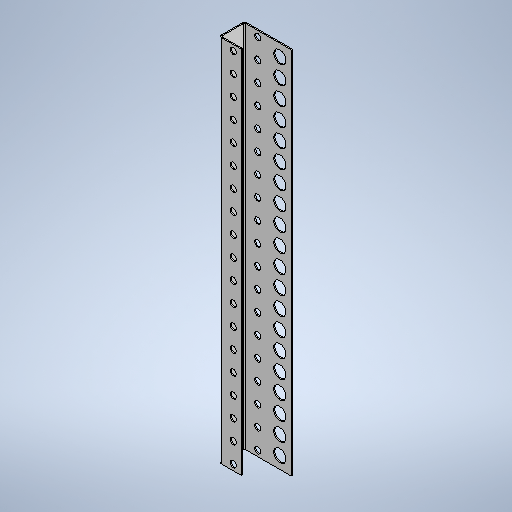
# Autodesk Inventor part: DMF 01 12 wheel pin
Saved by Autodesk Inventor 2026.2 (Build 302298010, 298A)
## iProperties
Created: 2024-04-30
Part Number: DMF 01 12 wheel pin
Material: Generic
Document SubType Name: Sheet Metal
Designer: admin
Density: 1 g/cm^3
Sheet Metal Rule: Default
Appearance: Default
Sheet Metal Width: 163,048 mm
Sheet Metal Length: 650,000 mm
Sheet Metal Area: 105981,061 mm^2
Stock Number: Барабан_Сектор_Усилителя
Flat Pattern Width: 16.3048 cm
Flat Pattern Length: 65 cm
Flat Pattern Area: 1059.81 cm^2
wheel_pin_L: 290,000 mm
wheel_pin_h: 25,000 mm
wheel_pin_Angle: 11,00 deg
Author: pokla
Autodesk Inventor part; units mm, degrees
ref_plane "YZ Plane" through (0, 0, 0) normal (1, 0, 0) x (0, 1, 0)
ref_plane "XZ Plane" through (0, 0, 0) normal (0, 1, 0) x (-1, 0, 0)
ref_plane "XY Plane" through (0, 0, 0) normal (0, 0, 1) x (1, 0, 0)
sketch "Sketch1" plane through (0, 0, 0) normal (0, 0, 1) x (1, 0, 0)
  line L0 (-42.5, 650) -> (42.5, 650)
  line L1 (42.5, 650) -> (42.5, 0)
  line L2 (42.5, 0) -> (-42.5, 0)
  line L3 (-42.5, 0) -> (-42.5, 650)
  point P0 (0, 0)
  point P1 (0, 0)
  point P2 (0, 0)
  point P3 (0, 0)
  point P4 (0, 0)
  dimension "d27" = 85
  dimension "d45" = 650
  measures "d27" distance of L1.end L2.end
  measures "d45" distance of L0.end L1.end
extrude "Plate1" add sketch "Sketch1" against normal blind 2
sketch "Sketch5" plane through (-40.5, 0, -2) normal (-1, 0, 0) x (0, -1, 0)
  line L0 (-650, 0) -> (0, 0)
  line L1 (0, 0) -> (0, 45)
  line L2 (0, 45) -> (-650, 45)
  line L3 (-650, 45) -> (-650, 0)
  constraints: 6 end point, 1 horizontal, 1 perpendicular, 1 vertical
edge flange "Flange2" height 45 angle 90 thickness 2 bend radius 2 thickness toward (-1, 0, 0) relief tear relief width 2 relief depth 1 edges at (-42.5, 325, 0) wall of the first edge with corners at (-40.5, 650, -2) (-40.5, 0, -2) (-40.5, 0, 43) (-40.5, 650, 43)
bend "Bend3"
corner "Corner2"
sketch "Sketch6" plane through (-42.5, 0, 41) normal (0, 0, 1) x (1, 0, 0)
  line L0 (0, 650) -> (0, 0)
  line L1 (0, 0) -> (40, 0)
  line L2 (40, 0) -> (40, 650)
  line L3 (40, 650) -> (0, 650)
  constraints: 6 end point, 1 horizontal, 1 perpendicular, 1 vertical
edge flange "Flange3" height 40 angle 90 thickness 2 bend radius 2 thickness toward (0, 0, 1) relief tear relief width 2 relief depth 1 edges at (-40.5, 325, 43) wall of the first edge with corners at (-42.5, 650, 41) (-42.5, 0, 41) (-2.5, 0, 41) (-2.5, 650, 41)
bend "Bend4"
corner "Corner3"
sketch "Sketch7" plane through (0, 0, 0) normal (0, 0, 1) x (1, 0, 0)
  circle A0 centre (21.5, 21.0949) radius 11
  circle A1 centre (-17.5, 10) radius 5.5
  line L0 (-38.5, 0) -> (-38.5, 650) construction
  line L1 (42.5, 650) -> (-38.5, 650) projected
  line L2 (42.5, 0) -> (42.5, 650) construction
  line L3 (-38.5, 0) -> (42.5, 0) projected
  line L4 (-38.5, 650) -> (-38.5, 0) construction
  line L5 (-2.5, 0) -> (-38.5, 0) projected
  line L6 (-2.5, 650) -> (-2.5, 0) construction
  line L7 (-38.5, 650) -> (-2.5, 650) projected
  circle A2 centre (-17.5, 45) radius 5.5
  circle A3 centre (-17.5, 80) radius 5.5
  circle A4 centre (-17.5, 115) radius 5.5
  circle A5 centre (-17.5, 150) radius 5.5
  circle A6 centre (-17.5, 185) radius 5.5
  circle A7 centre (-17.5, 220) radius 5.5
  circle A8 centre (-17.5, 255) radius 5.5
  circle A9 centre (-17.5, 290) radius 5.5
  circle A10 centre (-17.5, 325) radius 5.5
  circle A11 centre (-17.5, 360) radius 5.5
  circle A12 centre (-17.5, 395) radius 5.5
  circle A13 centre (-17.5, 430) radius 5.5
  circle A14 centre (-17.5, 465) radius 5.5
  circle A15 centre (-17.5, 500) radius 5.5
  circle A16 centre (-17.5, 535) radius 5.5
  circle A17 centre (-17.5, 570) radius 5.5
  circle A18 centre (-17.5, 605) radius 5.5
  circle A19 centre (-17.5, 640) radius 5.5
  circle A20 centre (21.5, 53.0949) radius 11
  circle A21 centre (21.5, 85.0949) radius 11
  circle A22 centre (21.5, 117.0949) radius 11
  circle A23 centre (21.5, 149.0949) radius 11
  circle A24 centre (21.5, 181.0949) radius 11
  circle A25 centre (21.5, 213.0949) radius 11
  circle A26 centre (21.5, 245.0949) radius 11
  circle A27 centre (21.5, 277.0949) radius 11
  circle A28 centre (21.5, 309.0949) radius 11
  circle A29 centre (21.5, 341.0949) radius 11
  circle A30 centre (21.5, 373.0949) radius 11
  circle A31 centre (21.5, 405.0949) radius 11
  circle A32 centre (21.5, 437.0949) radius 11
  circle A33 centre (21.5, 469.0949) radius 11
  circle A34 centre (21.5, 501.0949) radius 11
  circle A35 centre (21.5, 533.0949) radius 11
  circle A36 centre (21.5, 565.0949) radius 11
  circle A37 centre (21.5, 597.0949) radius 11
  circle A38 centre (21.5, 629.0949) radius 11
  point P0 (0, 0)
  dimension "d71" = 22
  dimension "d72" = 11
  dimension "d74" = 15
  dimension "d75" = 10
  dimension "d78" = 35
  dimension "d83" = 10
  dimension "d84" = 21
  dimension "d87" = 32
  constraints: 39 centre point, 2 vertical, 74 other
  measures "d71" diameter of A0
  measures "d72" diameter of A1
  measures "d74" distance from line of L6 A1.centre
  measures "d75" distance from line of L3 A1.centre
  measures "d78" distance of A1.centre A2.centre
  measures "d83" distance from line of A19.centre L7
  measures "d84" distance from line of L2 A0.centre
  measures "d87" distance of A0.centre A20.centre
extrude "Extrusion2" cut sketch "Sketch7" along normal through all both and the other way through all
fillet "Fillet1" radius 2 4 edges at (-2.5, 650, 42) (42.5, 650, -1) (-2.5, 0, 42) (42.5, 0, -1)
equation "\"d15\" = Thickness"
equation "\"d51\" = BendReliefWidth"
equation "\"d52\" = BendReliefDepth"
equation "\"d53\" = MinimumRemnant"
equation "\"d54\" = TransitionRadius"
equation "\"d57\" = BendRadius"
equation "\"d58\" = CornerReliefSize"
equation "\"d59\" = GapSize"
equation "\"d60\" = JacobiRadiusSize"
equation "\"d61\" = BendReliefWidth"
equation "\"d62\" = BendReliefDepth"
equation "\"d63\" = MinimumRemnant"
equation "\"d64\" = TransitionRadius"
equation "\"d67\" = BendRadius"
equation "\"d68\" = CornerReliefSize"
equation "\"d69\" = GapSize"
equation "\"d70\" = JacobiRadiusSize"
equation "\"BendRadius\" = Thickness"
equation "\"BendReliefWidth\" = Thickness"
equation "\"BendReliefDepth\" = 0.5 * Thickness"
equation "\"CornerReliefSize\" = 4 * Thickness"
equation "\"MinimumRemnant\" = 2 * Thickness"
equation "\"TransitionRadius\" = BendRadius"
equation "\"JacobiRadiusSize\" = BendRadius"
equation "\"GapSize\" = Thickness"
equation "\"wheel_pin_h\" = 25"
equation "\"wheel_pin_Angle\" = 11deg"
equation "\"Thickness\" = 2"
body "Solid1"
